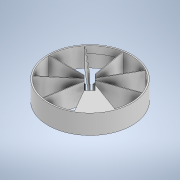
# Autodesk Inventor part: g
Saved by Autodesk Inventor 2022 (Build 260153000, 153)
## iProperties
Created: 2023-03-15
Part Number: g
Material: Типовые
Document SubType Name: Modeling
Designer: lrnto01
Density: 1 g/cm^3
Appearance: По умолчанию
Author: lrnto01
Autodesk Inventor part; units mm, degrees
ref_plane "YZ Plane" through (0, 0, 0) normal (1, 0, 0) x (0, 1, 0)
ref_plane "XZ Plane" through (0, 0, 0) normal (0, 1, 0) x (-1, 0, 0)
ref_plane "XY Plane" through (0, 0, 0) normal (0, 0, 1) x (1, 0, 0)
sketch "Эскиз1" plane through (0, 0, 0) normal (0, 1, 0) x (-1, 0, 0)
  circle A0 centre (0, 0) radius 65
  line L0 (0.731, 1.266) -> (11.4319, 61.9541)
  line L1 (-59.0278, -22.0164) -> (-1.1199, -0.9397)
  line L2 (-1.1199, -0.9397) -> (-31.932, -54.3079)
  line L3 (-0.2539, -1.4397) -> (10.4471, -62.1278)
  line L4 (1.3737, -0.5) -> (62.998, -0.5)
  line L5 (11.4319, -61.9541) -> (0.731, -1.266)
  line L6 (1.3737, 0.5) -> (48.5807, 40.1113)
  line L7 (48.5807, -40.1113) -> (1.3737, -0.5)
  line L8 (62.998, 0.5) -> (1.3737, 0.5)
  line L9 (47.9379, 40.8774) -> (0.731, 1.266)
  line L10 (-0.2539, 1.4397) -> (-31.066, 54.8079)
  line L11 (10.4471, 62.1278) -> (-0.2539, 1.4397)
  line L12 (-1.1199, 0.9397) -> (-59.0278, 22.0164)
  line L13 (-31.932, 54.3079) -> (-1.1199, 0.9397)
  line L14 (-1.4619, 0) -> (-59.3698, -21.0767)
  line L15 (-31.066, -54.8079) -> (-0.2539, -1.4397)
  line L16 (0.731, -1.266) -> (47.9379, -40.8774)
  line L17 (-59.3698, 21.0767) -> (-1.4619, 0)
  arc A1 (62.998, 0.5) -> (48.5807, 40.1113) centre (0, 0) ccw
  arc A2 (47.9379, 40.8774) -> (11.4319, 61.9541) centre (0, 0) ccw
  arc A3 (10.4471, 62.1278) -> (-31.066, 54.8079) centre (0, 0) ccw
  arc A4 (-31.932, 54.3079) -> (-59.0278, 22.0164) centre (0, 0) ccw
  arc A5 (-59.3698, 21.0767) -> (-59.3698, -21.0767) centre (0, 0) ccw
  arc A6 (-59.0278, -22.0164) -> (-31.932, -54.3079) centre (0, 0) ccw
  arc A7 (-31.066, -54.8079) -> (10.4471, -62.1278) centre (0, 0) ccw
  arc A8 (11.4319, -61.9541) -> (47.9379, -40.8774) centre (0, 0) ccw
  arc A9 (48.5807, -40.1113) -> (62.998, -0.5) centre (0, 0) ccw
  dimension "d1" = 130
  constraints: 36 end point, 18 point on circle, 10 centre point, 9 parallel, 2 coincident, 1 horizontal
  measures "d1" diameter of A0
extrude "Выдавливание1" add sketch "Эскиз1" along normal blind 2 contours A0 | L12 A4 L13
sketch "Эскиз2" plane through (0, 2, 0) normal (0, 1, 0) x (1, 0, 0)
  line L0 (-4.2111, 3.5379) -> (0.0316, 7.7806)
  line L1 (-4.2111, 3.5379) -> (1.7889, 3.5379) construction
  line L2 (-4.2111, 3.5379) -> (-8.4537, -0.7047)
  line L3 (-4.2111, 3.5379) -> (1.7889, 3.5379) construction
  line L4 (0.0316, 7.7806) -> (16.295, -8.4829)
  line L5 (0.0316, 7.7806) -> (23.0316, 7.7806) construction
  line L6 (16.295, -8.4829) -> (7.8098, -16.9682)
  line L7 (7.8098, -16.9682) -> (-8.4537, -0.7047)
  circle A0 centre (0, 0) radius 65
  line L8 (-62.998, -0.5) -> (-1.3737, -0.5) projected
  line L9 (-1.3737, -0.5) -> (-48.5807, -40.1113) projected
  line L10 (-62.998, -0.5) -> (-8.249, -0.5)
  line L11 (-47.9379, -40.8774) -> (-0.731, -1.266) projected
  line L12 (-5.3347, -3.8237) -> (-48.5807, -40.1113)
  line L13 (-0.731, -1.266) -> (-11.4319, -61.9541) projected
  line L14 (-47.9379, -40.8774) -> (-4.6249, -4.5335)
  arc A1 (-47.9379, -40.8774) -> (-11.4319, -61.9541) centre (0, 0) ccw projected
  line L15 (-1.8044, -7.354) -> (-11.4319, -61.9541)
  line L16 (-11.4319, -61.9541) -> (-11.4319, -61.9541)
  line L17 (-10.4471, -62.1278) -> (0.2539, -1.4397) projected
  line L18 (0.2539, -1.4397) -> (31.066, -54.8079) projected
  line L19 (8.7033, -16.0746) -> (31.066, -54.8079)
  arc A2 (59.3698, -21.0767) -> (59.3698, 21.0767) centre (0, 0) ccw projected
  line L20 (1.4619, 0) -> (59.3698, 21.0767) projected
  line L21 (59.3698, -21.0767) -> (11.4461, -3.634)
  line L22 (6.1176, 1.6945) -> (59.3698, 21.0767)
  arc A3 (59.0278, 22.0164) -> (31.932, 54.3079) centre (0, 0) ccw projected
  line L23 (59.0278, 22.0164) -> (1.1199, 0.9397) projected
  line L24 (59.0278, 22.0164) -> (5.3374, 2.4747)
  line L25 (1.1199, 0.9397) -> (31.932, 54.3079) projected
  line L26 (3.2255, 4.5867) -> (31.932, 54.3079)
  line L27 (31.066, 54.8079) -> (0.2539, 1.4397) projected
  line L28 (0.2539, 1.4397) -> (-10.4471, 62.1278) projected
  arc A4 (31.066, 54.8079) -> (-10.4471, 62.1278) centre (0, 0) ccw projected
  line L29 (-10.4471, 62.1278) -> (-10.4471, 62.1278)
  line L30 (-11.4319, 61.9541) -> (-0.731, 1.266) projected
  arc A5 (-11.4319, 61.9541) -> (-47.9379, 40.8774) centre (0, 0) ccw projected
  line L31 (-3.4385, 3.5379) -> (-47.9379, 40.8774)
  line L32 (-47.9379, 40.8774) -> (-47.9379, 40.8774)
  line L33 (-1.3737, 0.5) -> (-62.998, 0.5) projected
  line L34 (-4.5684, 3.1806) -> (-48.5807, 40.1113)
  line L35 (-0.731, 1.266) -> (-47.9379, 40.8774) projected
  line L36 (-48.5807, 40.1113) -> (-1.3737, 0.5) projected
  arc A6 (-48.5807, 40.1113) -> (-62.998, 0.5) centre (0, 0) ccw projected
  line L37 (-7.249, 0.5) -> (-62.998, 0.5)
  arc A7 (-62.998, -0.5) -> (-48.5807, -40.1113) centre (0, 0) ccw
  arc A8 (-47.9379, -40.8774) -> (-11.4319, -61.9541) centre (0, 0) ccw
  arc A9 (-10.4471, -62.1278) -> (31.066, -54.8079) centre (0, 0) ccw
  arc A10 (59.3698, -21.0767) -> (-10.4471, 62.1278) centre (0, 0) ccw
  arc A11 (-11.4319, 61.9541) -> (-47.9379, 40.8774) centre (0, 0) ccw
  arc A12 (-48.5807, 40.1113) -> (-62.998, 0.5) centre (0, 0) ccw
  line L38 (-0.7299, 7.0191) -> (-10.4471, 62.1278)
  line L39 (31.066, 54.8079) -> (2.4934, 5.3187)
  point P0 (-8.249, -0.5)
  point P1 (-7.249, 0.5)
  point P2 (-3.8586, 3.8904)
  point P3 (-1.5932, 6.1558)
  point P4 (-0.7299, 7.0191)
  point P5 (5.3374, 2.4747)
  point P6 (6.1176, 1.6945)
  point P7 (-0.9412, -8.2172)
  point P8 (-1.8044, -7.354)
  point P9 (-4.6249, -4.5335)
  point P10 (-5.3347, -3.8237)
  dimension "d7" = 6
  dimension "d8" = 45
  dimension "d10" = 6
  dimension "d11" = 135
  dimension "d12" = 23
  dimension "d13" = 45
  dimension "d14" = 12
  constraints: 52 end point, 16 point on circle, 14 point on line, 7 centre point, 5 horizontal, 4 collinear, 3 equal length, 3 tangent, 2 coincident, 2 parallel, 2 perpendicular, 3 other
  measures "d7" distance of L0.start L0.end
  measures "d8" angle of L1 L0
  measures "d10" distance of L0.start L2.end
  measures "d11" angle of L2 L3
  measures "d12" distance of L0.end L4.end
  measures "d13" angle of L4 L5
  measures "d14" distance of L4.end L6.end
extrude "Выдавливание2" add sketch "Эскиз2" along normal blind 17 contours L27 A10 L25 L4 | L23 A10 L20 L4 | A0
sketch "Эскиз3" plane through (0, 19, 0) normal (0, 1, 0) x (1, 0, 0)
  line L0 (59.3698, -21.0767) -> (1.4619, 0) projected
  line L1 (5.3374, 2.4747) -> (6.1176, 1.6945) projected
  line L2 (11.4461, -3.634) -> (6.1176, 1.6945)
  line L3 (3.2255, 4.5867) -> (2.4934, 5.3187) projected
  line L4 (6.1176, 1.6945) -> (2.4934, 5.3187)
  line L5 (2.4934, 5.3187) -> (0, 7.8122)
  line L6 (-0.7299, 7.0191) -> (-1.5932, 6.1558) projected
  line L7 (-3.8586, 3.8904) -> (-47.9379, 40.8774) projected
  line L8 (-62.998, -0.5) -> (-8.249, -0.5) projected
  line L9 (16.295, -8.4829) -> (11.4461, -3.634) projected
  line L10 (11.4461, -3.634) -> (16.295, -8.4829)
  line L11 (0.2539, -1.4397) -> (8.7033, -16.0746) projected
  line L12 (-8.249, -0.5) -> (-7.249, 0.5) projected
  line L13 (-1.3737, -0.5) -> (-5.3347, -3.8237) projected
  line L14 (-5.3347, -3.8237) -> (-4.6249, -4.5335) projected
  line L15 (-5.3347, -3.8237) -> (-4.6249, -4.5335)
  line L16 (-4.6249, -4.5335) -> (-8.4639, -0.6945)
  line L17 (-4.6249, -4.5335) -> (7.8098, -16.9682)
  line L18 (8.7033, -16.0746) -> (16.295, -8.4829) projected
  line L19 (-8.4639, -0.6945) -> (-11.9994, 2.841)
  line L20 (-11.9994, 2.841) -> (-3.5142, 11.3263)
  line L21 (-3.5142, 11.3263) -> (0, 7.8122)
  line L22 (16.295, -8.4829) -> (19.6141, -11.802)
  line L23 (19.6141, -11.802) -> (11.1446, -20.303)
  line L24 (11.1446, -20.303) -> (7.8098, -16.9682)
  circle A0 centre (0, 0) radius 65
  line L25 (-7.249, 0.5) -> (-62.998, 0.5) projected
  line L26 (-9.6584, 0.5) -> (-62.998, 0.5)
  line L27 (-5.3347, -3.8237) -> (-48.5807, -40.1113) projected
  line L28 (-8.6584, -0.5) -> (-5.3347, -3.8237)
  arc A1 (-62.998, -0.5) -> (-48.5807, -40.1113) centre (0, 0) ccw projected
  line L29 (-5.3347, -3.8237) -> (-48.5807, -40.1113)
  line L30 (-47.9379, -40.8774) -> (-4.6249, -4.5335) projected
  line L31 (-47.9379, -40.8774) -> (-4.6249, -4.5335)
  line L32 (-1.8044, -7.354) -> (-0.9412, -8.2172) projected
  line L33 (-4.6249, -4.5335) -> (-1.8044, -7.354)
  arc A2 (-47.9379, -40.8774) -> (-11.4319, -61.9541) centre (0, 0) ccw projected
  line L34 (-1.8044, -7.354) -> (-11.4319, -61.9541)
  line L35 (-10.4471, -62.1278) -> (-0.9412, -8.2172) projected
  line L36 (-10.9395, -62.0409) -> (-10.4471, -62.1278)
  line L37 (-10.4471, -62.1278) -> (-0.9412, -8.2172)
  line L38 (-0.9412, -8.2172) -> (11.1446, -20.303)
  line L39 (-0.9412, -8.2172) -> (11.1446, -20.303)
  line L40 (8.7033, -16.0746) -> (31.066, -54.8079) projected
  line L41 (11.1446, -20.303) -> (31.066, -54.8079)
  line L42 (11.4461, -3.634) -> (6.1176, 1.6945)
  line L43 (1.4619, 0) -> (59.3698, 21.0767) projected
  line L44 (59.0278, 22.0164) -> (5.3374, 2.4747) projected
  line L45 (59.0278, 22.0164) -> (5.3374, 2.4747)
  line L46 (5.3374, 2.4747) -> (3.2255, 4.5867)
  line L47 (3.2255, 4.5867) -> (31.932, 54.3079)
  line L48 (31.066, 54.8079) -> (0.2539, 1.4397) projected
  line L49 (31.066, 54.8079) -> (2.4934, 5.3187)
  line L50 (0, 7.8122) -> (0, 62.998)
  arc A3 (31.066, 54.8079) -> (-10.4471, 62.1278) centre (0, 0) ccw projected
  line L51 (-10.4471, 62.1278) -> (-1.056, 8.8681)
  line L52 (0.2539, 1.4397) -> (-10.4471, 62.1278) projected
  line L53 (-11.4319, 61.9541) -> (-0.731, 1.266) projected
  line L54 (-2.2888, 10.1009) -> (-11.4319, 61.9541)
  line L55 (31.066, -54.8079) -> (31.0696, -54.8035)
  line L56 (59.3661, -21.0811) -> (59.3698, -21.0767)
  arc A4 (59.3661, -21.0811) -> (59.3679, 21.0761) centre (0, 0) ccw
  arc A5 (59.0259, 22.0158) -> (31.931, 54.3062) centre (0, 0) ccw
  arc A6 (31.065, 54.8062) -> (-10.4467, 62.1258) centre (0, 0) ccw
  arc A7 (-11.4315, 61.9522) -> (-47.9364, 40.8761) centre (0, 0) ccw
  arc A8 (-62.996, -0.5) -> (-48.5792, -40.11) centre (0, 0) ccw
  arc A9 (-47.9364, -40.8761) -> (-11.4315, -61.9522) centre (0, 0) ccw
  arc A10 (-10.4467, -62.1258) -> (31.0696, -54.8035) centre (0, 0) ccw
  arc A11 (-48.5807, 40.1113) -> (-62.998, 0.5) centre (0, 0) ccw projected
  line L57 (-62.998, 0.5) -> (-9.6584, 0.5)
  line L58 (-11.9994, 2.841) -> (-8.4243, 6.4161)
  arc A12 (-48.5807, 40.1113) -> (-62.998, 0.5) centre (0, 0) ccw
  line L59 (-48.5807, 40.1113) -> (-1.3737, 0.5) projected
  line L60 (-8.4243, 6.4161) -> (-48.5807, 40.1113)
  line L61 (-48.5807, 40.1113) -> (-8.4243, 6.4161)
  line L62 (-11.9994, 2.841) -> (-8.4243, 6.4161)
  line L63 (-11.9994, 2.841) -> (-9.6584, 0.5)
  line L64 (-62.998, 0.5) -> (-9.6584, 0.5)
  point P0 (-10.4467, -62.1258)
  point P1 (-7.7145, 7.126)
  point P2 (-11.4315, 61.9522)
  point P3 (59.3679, -21.0761)
  point P4 (31.065, -54.8062)
  dimension "d18" = 12
  constraints: 82 end point, 24 point on line, 18 point on circle, 17 collinear, 9 centre point, 3 perpendicular, 2 coincident, 2 horizontal, 1 concentric, 1 parallel, 1 vertical
  measures "d18" distance of L19.end L20.end
extrude "Выдавливание3" add sketch "Эскиз3" along normal blind 11
